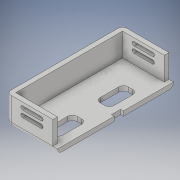
# Autodesk Inventor part: Power_Supply_Shroud
Saved by Autodesk Inventor 2019.4 (Build 234330000, 330)
## iProperties
Created: 2020-03-13
Part Number: Power_Supply_Shroud
Material: Generic
Document SubType Name: Modeling
Designer: Jorian Bruslind
Density: 1 g/cm^3
Appearance: Default
Author: Jorian Bruslind
Autodesk Inventor part; units mm, degrees
ref_plane "YZ Plane" through (0, 0, 0) normal (1, 0, 0) x (0, 1, 0)
ref_plane "XZ Plane" through (0, 0, 0) normal (0, 1, 0) x (-1, 0, 0)
ref_plane "XY Plane" through (0, 0, 0) normal (0, 0, 1) x (1, 0, 0)
sketch "Sketch1" plane through (0, 0, 0) normal (0, 1, 0) x (-1, 0, 0)
  line L0 (0, 0) -> (45, 0)
  line L1 (45, 0) -> (45, -115)
  line L2 (45, -115) -> (0, -115)
  line L3 (0, -115) -> (0, 0)
  line L4 (50, -120) -> (50, 5)
  line L5 (50, 5) -> (-5, 5)
  line L6 (-5, 5) -> (-5, -120)
  line L7 (-5, -120) -> (50, -120)
  dimension "d0" = 45
  dimension "d1" = 115
  dimension "d2" = 5
  constraints: 16 end point, 4 parallel, 2 perpendicular, 1 horizontal, 3 other
  measures "d0" distance of L1.end L2.end
  measures "d1" distance of L0.end L1.end
  measures "d2" distance between parallel lines of L1 L4
extrude "Extrusion1" add sketch "Sketch1" along normal blind 5 contours L0 L1 L2 L3 | L7 L6 L5 L4
sketch "Sketch2" plane through (0, 5, 0) normal (0, 1, 0) x (1, 0, 0)
  line L0 (0, 0) -> (-45, 0)
  line L1 (-45, 0) -> (-45, 115)
  line L2 (-45, 115) -> (0, 115)
  line L3 (0, 115) -> (0, 0)
  line L4 (5, 120) -> (-50, 120)
  line L5 (-50, 120) -> (-50, -5)
  line L6 (-50, -5) -> (5, -5)
  line L7 (0, 115) -> (0, 120)
  line L8 (5, 120) -> (-50, 120) projected
  line L9 (0, 0) -> (0, -5)
  dimension "d5" = 45
  dimension "d6" = 115
  dimension "d7" = 5
  constraints: 18 end point, 3 parallel, 3 perpendicular, 3 point on line, 1 horizontal, 2 other
  measures "d5" distance of L1.end L2.end
  measures "d6" distance of L0.end L1.end
  measures "d7" distance between parallel lines of L2 L4
extrude "Extrusion2" add sketch "Sketch2" along normal blind 25 contours L9 L6 L5 L4 L7 L2 L1 L0
sketch "Sketch3" plane through (-50, 0, 5) normal (0, 0, 1) x (1, 0, 0)
  line L0 (5, 30) -> (50, 30) projected
  line L1 (27.5, 30) -> (27.5, 24.5)
  line L2 (17.5, 24.5) -> (37.5, 24.5) construction
  line L3 (17.5, 22.5) -> (37.5, 22.5)
  line L4 (37.5, 26.5) -> (17.5, 26.5)
  arc A0 (17.5, 26.5) -> (17.5, 22.5) centre (17.5, 24.5) ccw
  arc A1 (37.5, 22.5) -> (37.5, 26.5) centre (37.5, 24.5) ccw
  line L5 (27.5, 24.5) -> (47.5, 24.5) construction
  point P0 (50, 0)
  dimension "d10" = 5.5
  dimension "d11" = 10
  dimension "d12" = 0
  dimension "d13" = 4
  constraints: 12 end point, 4 point on circle, 4 tangent, 2 centre point, 2 horizontal, 2 midpoint, 1 collinear, 1 parallel, 1 vertical
  measures "d10" distance of L1.start L1.end
  measures "d11" distance of L1.end L2.end
  measures "d12" distance between parallel lines of L2 L5
  measures "d13" diameter of A1
extrude "Extrusion3" cut sketch "Sketch3" against normal blind 125
sketch "Sketch4" plane through (0, 5, 0) normal (0, 1, 0) x (1, 0, 0)
  line L0 (-45, 0) -> (-45, 115) projected
  line L1 (-45, 0) -> (-20, 0)
  line L2 (-45, 0) -> (0, 0) projected
  line L3 (-20, 0) -> (-20, 6)
  line L4 (-20, 6) -> (-5, 6)
  line L5 (-5, 6) -> (-5, 36)
  line L6 (-5, 36) -> (-20, 36)
  line L7 (-20, 36) -> (-20, 6)
  line L8 (-5, 91) -> (-20, 91)
  line L9 (-5, 61) -> (-5, 91)
  line L10 (-20, 91) -> (-20, 61)
  line L11 (-20, 61) -> (-5, 61)
  dimension "d16" = 25
  dimension "d17" = 6
  dimension "d18" = 15
  dimension "d19" = 30
  dimension "d22" = 55
  constraints: 20 end point, 2 parallel, 2 vertical, 1 horizontal, 1 perpendicular, 1 point on line, 8 other
  measures "d16" distance of L0.start L1.end
  measures "d17" distance of L1.end L3.end
  measures "d18" distance of L6.end L5.end
  measures "d19" distance of L5.end L4.end
  measures "d22" distance of L5.end L8.start
extrude "Extrusion4" cut sketch "Sketch4" against normal blind 5
fillet "Fillet1" radius 5 5 edges at (-22.5, 0, 5) (-22.5, 0, -120) (-50, 0, -57.5) (-50, 15, 5) (-50, 15, -120)
fillet "Fillet2" radius 5 8 edges at (-20, 2.5, -6) (-5, 2.5, -36) (-5, 2.5, -91) (-20, 2.5, -36) (-20, 2.5, -91) (-5, 2.5, -6) (-5, 2.5, -61) (-20, 2.5, -61)
pattern_linear "Rectangular Pattern1" count 2 spacing 7 along (0, -1, 0) of "Extrusion3"
sketch "Sketch5" plane through (5, 0, 0) normal (1, 0, 0) x (0, 0, -1)
  line L0 (61, 0) -> (61, 5) projected
  line L1 (0, 0) -> (61, 0)
  line L2 (61, 0) -> (61, 5)
  line L3 (61, 5) -> (66, 5)
  line L4 (66, 5) -> (66, 0)
  line L5 (66, 0) -> (61, 0)
  line L6 (61, 5) -> (61, 0)
  line L7 (61, 0) -> (56, 0)
  line L8 (56, 0) -> (56, 5)
  line L9 (56, 5) -> (61, 5)
  dimension "d34" = 5
  dimension "d35" = 5
  constraints: 18 end point, 4 parallel, 3 perpendicular, 1 horizontal, 1 vertical
  measures "d34" distance of L0.end L3.end
  measures "d35" distance of L0.start L7.end
extrude "Extrusion5" cut sketch "Sketch5" against normal blind 3
body "Solid1"
